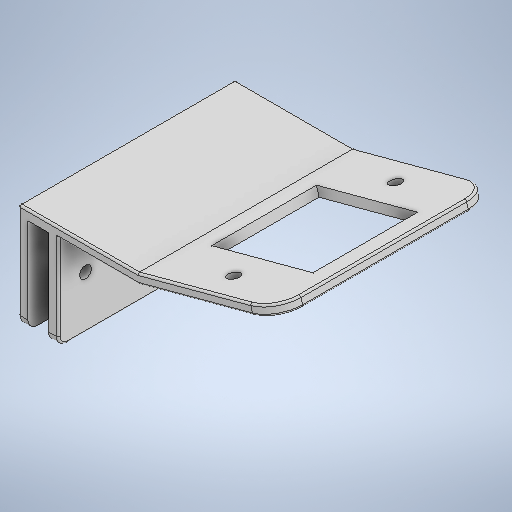
# Autodesk Inventor part: CamMountThrify
Saved by Autodesk Inventor 2025 (Build 290162000, 162)
## iProperties
Created: 2025-03-11
Part Number: CamMountThrify
Material: Generic
Document SubType Name: Modeling
Designer: john
Density: 1 g/cm^3
Appearance: Default
Author: john
Autodesk Inventor part; units mm, degrees
ref_plane "YZ Plane" through (0, 0, 0) normal (1, 0, 0) x (0, 1, 0)
ref_plane "XZ Plane" through (0, 0, 0) normal (0, 1, 0) x (-1, 0, 0)
ref_plane "XY Plane" through (0, 0, 0) normal (0, 0, 1) x (1, 0, 0)
sketch "Sketch1" plane through (0, 0, 0) normal (0, 0, 1) x (1, 0, 0)
  line L0 (0, 0) -> (-6.5, 0)
  line L1 (-6.5, 0) -> (-6.5, -30)
  line L2 (-6.5, 0) -> (23.5, 0) construction
  line L3 (0, 0) -> (0, -30)
  line L4 (3, 0) -> (3, -30)
  line L5 (0, 3) -> (-9.5, 3)
  line L6 (-9.5, 3) -> (-9.5, -30)
  line L7 (3, -30) -> (0, -30)
  line L8 (-6.5, -30) -> (-9.5, -30)
  line L9 (28.4, 0) -> (71.8667, 11.6469)
  line L10 (28.4, 0) -> (73.4, 0) construction
  line L11 (28.4, 0) -> (3, 0)
  line L12 (0, 3) -> (28.005, 3)
  line L13 (71.0902, 14.5446) -> (28.005, 3)
  line L14 (71.8667, 11.6469) -> (71.0902, 14.5446)
  dimension "d0" = 6.5
  dimension "d1" = 30
  dimension "d2" = 90
  dimension "d3" = 30
  dimension "d4" = 3
  dimension "d5" = 3
  dimension "d6" = 25.4
  dimension "d7" = 45
  dimension "d8" = 15
  constraints: 30 end point, 6 horizontal, 2 equal length, 2 vertical, 1 collinear, 1 parallel, 1 perpendicular, 1 other
  measures "d0" distance of L0.start L0.end
  measures "d1" distance of L0.end L1.end
  measures "d2" angle of L1 L2
  measures "d3" distance of L3.start L3.end
  measures "d4" distance between parallel lines of L3 L4
  measures "d5" distance between parallel lines of L0 L5
  measures "d6" distance of L4.start L9.start
  measures "d7" distance of L9.start L9.end
  measures "d8" angle of L10 L9
extrude "Extrusion1" add sketch "Sketch1" along normal blind 68
sketch "Sketch2" plane through (71.8667, 11.6469, 0) normal (0.2588, -0.9659, 0) x (0.9659, 0.2588, 0)
  line L0 (0, 0) -> (-44.605, 0) construction
  line L1 (-22.3025, 0) -> (-22.3025, 68) construction
  line L2 (0, 68) -> (-44.605, 68) construction
  circle A0 centre (-22.3025, 34) radius 25.4 construction
  circle A1 centre (-22.3025, 8.6) radius 1.85
  circle A2 centre (-22.3025, 59.4) radius 1.85
  line L3 (-5.8525, 50.45) -> (-38.7525, 50.45)
  line L4 (-38.7525, 50.45) -> (-38.7525, 17.55)
  line L5 (-38.7525, 17.55) -> (-5.8525, 17.55)
  line L6 (-5.8525, 17.55) -> (-5.8525, 50.45)
  line L7 (-5.8525, 50.45) -> (-38.7525, 17.55) construction
  line L8 (-38.7525, 50.45) -> (-5.8525, 17.55) construction
  point P0 (-72.4323, 0)
  dimension "d12" = 50.8
  dimension "d13" = 3.7
  dimension "d14" = 3.7
  dimension "d15" = 32.9
  dimension "d16" = 32.9
  constraints: 14 end point, 5 midpoint, 3 centre point, 2 coincident, 2 parallel, 2 point on circle, 2 point on line, 1 horizontal, 1 perpendicular
  measures "d12" diameter of A0
  measures "d13" diameter of A1
  measures "d14" diameter of A2
  measures "d15" distance of L5.end L4.end
  measures "d16" distance of L4.end L3.end
extrude "Extrusion2" cut sketch "Sketch2" against normal blind 68
sketch "Sketch3" plane through (-9.5, -30, 0) normal (-1, 0, 0) x (0, 0, 1)
  line L0 (0, 33) -> (0, 0) construction
  line L1 (0, 16.5) -> (68, 16.5) construction
  line L2 (68, 33) -> (68, 0) construction
  circle A0 centre (34, 16.5) radius 1.85
  circle A1 centre (46.7, 16.5) radius 1.85
  circle A2 centre (21.3, 16.5) radius 1.85
  circle A3 centre (59.4, 16.5) radius 1.85
  circle A4 centre (8.6, 16.5) radius 1.85
  point P0 (0, 30)
  dimension "d19" = 3.7
  dimension "d22" = 12.7
  constraints: 5 centre point, 3 midpoint, 2 end point, 1 horizontal, 8 other
  measures "d19" diameter of A0
  measures "d22" distance of A0.centre A1.centre
extrude "Extrusion3" cut sketch "Sketch3" against normal blind 68
fillet "Fillet1" radius 8 2 edges at (71.4784, 13.0957, 0) (71.4784, 13.0957, 68)
fillet "Fillet2" radius 3 4 edges at (1.5, -30, 68) (-8, -30, 68) (1.5, -30, 0) (-8, -30, 0)
fillet "Fillet3" radius 0.6 25 edges at (-9.5, 3, 34) (-9.5, -29.1213, 67.1213) (-9.5, -30, 34) (-9.5, -29.1213, 0.8787) (-9.5, -12, 0) (-9.5, -12, 68) (9.2525, 3, 68) (9.2525, 3, 0) (68.8269, 13.9382, 2.3431) (71.0902, 14.5446, 34) (68.8269, 13.9382, 65.6569) (45.6839, 7.737, 68) (45.6839, 7.737, 0) (69.6034, 11.0404, 65.6569) (71.8667, 11.6469, 34) (69.6034, 11.0404, 2.3431) (46.2696, 4.7882, 0) (46.2696, 4.7882, 68) (15.7, 0, 68) (15.7, 0, 0) (3, -29.1213, 67.1213) (3, -13.5, 68) (3, -29.1213, 0.8787) (3, -13.5, 0) (3, -30, 34)
chamfer "Chamfer1" [suppressed]
body "Solid1"
